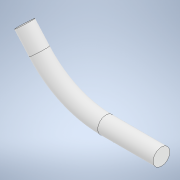
# Autodesk Inventor part: Landing_gear_pin
Saved by Autodesk Inventor 2021 (Build 250183000, 183)
## iProperties
Created: 2020-11-24
Part Number: Landing_gear_pin
Material: ABS Plastic
Document SubType Name: Modeling
Designer: Kanenas
Mass: 0.206529 g
Surface Area: 2.73922 cm^2
Volume: 0.194838 cm^3
Density: 1.06 g/cm^3
Appearance: Smooth - White
Author: Kanenas
Autodesk Inventor part; units mm, degrees
ref_plane "YZ Plane" through (0, 0, 0) normal (1, 0, 0) x (0, 1, 0)
ref_plane "XZ Plane" through (0, 0, 0) normal (0, 1, 0) x (-1, 0, 0)
ref_plane "XY Plane" through (0, 0, 0) normal (0, 0, 1) x (1, 0, 0)
sketch "Sketch1" plane through (0, 0, 0) normal (0, 0, 1) x (1, 0, 0)
  line L0 (0, 0) -> (10, 0)
  arc A0 (-12, 5.408) -> (0, 0) centre (0, 16.0176) ccw
  dimension "d3" = 10
  dimension "d4" = 12
  constraints: 2 end point, 2 point on circle, 1 centre point, 1 horizontal, 1 tangent
  measures "d3" distance of L0.start L0.end
  measures "d4" horizontal distance of L0.start A0.start
sketch "Sketch2" plane through (0, 0, 0) normal (1, 0, 0) x (0, 1, 0)
  circle A0 centre (0, 0) radius 1.5
  dimension "d0" = 3
  constraints: 1 centre point, 1 coincident
  measures "d0" diameter of A0
sweep "Sweep1" add profiles "Sketch2" path "Sketch1"
sketch "Sketch3" plane through (-12, 5.408, 0) normal (-0.6624, 0.7492, 0) x (0.7492, 0.6624, 0)
  circle A0 centre (0, 0) radius 1.5 projected
  point P0 (5.408, 0)
extrude "Extrusion1" add sketch "Sketch3" along normal blind 4
body "Solid1"
